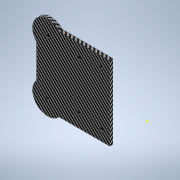
# Autodesk Inventor part: Power Distribution Board redo v2
Saved by Autodesk Inventor 2020.2 (Build 242310000, 310)
## iProperties
Created: 2020-08-30
Part Number: Power Distribution Board redo v2
Material: CFRP
Document SubType Name: Modeling
Designer: Krishna Makhija
Density: 1.43 g/cm^3
Appearance: Carbon Fiber
Author: Krishna Makhija
Autodesk Inventor part; units mm, degrees
ref_plane "YZ Plane" through (0, 0, 0) normal (1, 0, 0) x (0, 1, 0)
ref_plane "XZ Plane" through (0, 0, 0) normal (0, 1, 0) x (-1, 0, 0)
ref_plane "XY Plane" through (0, 0, 0) normal (0, 0, 1) x (1, 0, 0)
sketch "Sketch1" plane through (0, 0, 0) normal (0, 0, 1) x (1, 0, 0)
  point P0 (0, 0)
sketch "Sketch2" plane through (0, 0, 0) normal (0, 0, 1) x (1, 0, 0)
  line L0 (-100, -34.5) -> (-100, 34.5)
  circle A0 centre (-60, 22) radius 1.4998
  circle A1 centre (-60, -22) radius 1.4998
  circle A2 centre (-89.5, 25) radius 1.4998
  circle A3 centre (-89.5, -25) radius 1.4998
  circle A4 centre (-39.5, 25) radius 1.4998
  circle A5 centre (-39.5, -25) radius 1.4998
  circle A6 centre (-89.5, 25) radius 14.1598
  circle A7 centre (-89.5, -25) radius 14.1598
  line L1 (-32, 34.5) -> (-32, -34.5)
  line L2 (-32, 34.5) -> (-100, 34.5)
  line L3 (-32, -34.5) -> (-100, -34.5)
  point P0 (-100, 15.5)
  point P1 (-100, -15.5)
  point P2 (-79, -34.5)
  point P3 (-79, 34.5)
  constraints: 8 end point, 6 centre point, 2 coincident, 2 horizontal, 6 other
extrude "Extrusion1" add sketch "Sketch2" along normal blind 3
body "Solid1"
